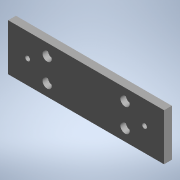
# Autodesk Inventor part: adapter_stage
Saved by Autodesk Inventor 2022 (Build 260153000, 153)
## iProperties
Part Number: adapter_stage
Material: Allgemein
Document SubType Name: Modellieren
Designer: Niclas
Appearance: Vorgabe
Author: Niclas
Autodesk Inventor part; units mm, degrees
ref_plane "YZ-Ebene" through (0, 0, 0) normal (1, 0, 0) x (0, 1, 0)
ref_plane "XZ-Ebene" through (0, 0, 0) normal (0, 1, 0) x (-1, 0, 0)
ref_plane "XY-Ebene" through (0, 0, 0) normal (0, 0, 1) x (1, 0, 0)
sketch "Skizze1" plane through (0, 0, 0) normal (0, 0, 1) x (1, 0, 0)
  line L0 (-200, 60) -> (0, 60)
  line L1 (0, 60) -> (0, 0)
  line L2 (0, 0) -> (-200, 0)
  line L3 (-200, 0) -> (-200, 60)
  dimension "d0" = 200
  dimension "d1" = 60
  constraints: 8 end point, 2 parallel, 1 coincident, 1 horizontal, 1 perpendicular
  measures "d0" distance of L0.start L0.end
  measures "d1" distance of L2.end L0.start
extrude "Extrusion1" add sketch "Skizze1" along normal blind 10
sketch "Skizze2" plane through (0, 0, 10) normal (0, 0, 1) x (1, 0, 0)
  circle A0 centre (-175, 30) radius 3.1
  circle A1 centre (-25, 30) radius 3.1
  line L0 (-200, 0) -> (0, 0) projected
  line L1 (0, 0) -> (0, 60) projected
  circle A2 centre (-150, 45) radius 3.1
  circle A3 centre (-50, 45) radius 3.1
  circle A4 centre (-150, 15) radius 3.1
  circle A5 centre (-50, 15) radius 3.1
  line L2 (0, 60) -> (-200, 60) projected
  dimension "d4" = 6.2
  dimension "d5" = 6.2
  dimension "d6" = 30
  dimension "d7" = 30
  dimension "d8" = 150
  dimension "d9" = 25
  dimension "d10" = 6.2
  dimension "d11" = 6.2
  dimension "d12" = 6.2
  dimension "d13" = 6.2
  dimension "d14" = 30
  dimension "d15" = 30
  dimension "d16" = 100
  dimension "d17" = 100
  dimension "d18" = 50
  dimension "d19" = 50
  dimension "d20" = 15
  dimension "d21" = 15
  constraints: 6 centre point
  measures "d4" diameter of A1
  measures "d5" diameter of A0
  measures "d6" distance from line of A0.centre L0
  measures "d7" distance from line of L0 A1.centre
  measures "d8" distance of A1.centre A0.centre
  measures "d9" distance from line of L1 A1.centre
  measures "d10" diameter of A2
  measures "d11" diameter of A3
  measures "d12" diameter of A5
  measures "d13" diameter of A4
  measures "d14" distance of A4.centre A2.centre
  measures "d15" distance of A5.centre A3.centre
  measures "d16" distance of A5.centre A4.centre
  measures "d17" distance of A3.centre A2.centre
  measures "d18" distance from line of L1 A3.centre
  measures "d19" distance from line of L1 A5.centre
  measures "d20" distance from line of L2 A3.centre
  measures "d21" distance from line of L2 A2.centre
extrude "Extrusion2" cut sketch "Skizze2" against normal blind 15
sketch "Skizze3" plane through (0, 0, 10) normal (0, 0, 1) x (1, 0, 0)
  circle A0 centre (-150, 45) radius 3.1 projected
  circle A1 centre (-150, 45) radius 6
  circle A2 centre (-150, 15) radius 3.1 projected
  circle A3 centre (-150, 15) radius 6
  circle A4 centre (-50, 45) radius 3.1 projected
  circle A5 centre (-50, 15) radius 3.1 projected
  circle A6 centre (-50, 15) radius 6
  circle A7 centre (-50, 45) radius 6
  point P0 (0, 0)
  dimension "d24" = 12
  dimension "d25" = 12
  dimension "d26" = 12
  dimension "d27" = 12
  constraints: 4 centre point, 4 coincident
  measures "d24" diameter of A1
  measures "d25" diameter of A3
  measures "d26" diameter of A6
  measures "d27" diameter of A7
extrude "Extrusion3" cut sketch "Skizze3" against normal blind 7 contours A1 | A3 | A5 | A6 | A7
sketch "Skizze4" plane through (0, 0, 0) normal (0, 0, -1) x (-1, 0, 0)
  circle A0 centre (175, 30) radius 3.1 projected
  circle A1 centre (175, 30) radius 6
  circle A2 centre (25, 30) radius 3.1 projected
  circle A3 centre (25, 30) radius 6
  point P0 (0, 0)
  dimension "d30" = 12
  dimension "d31" = 12
  constraints: 2 centre point, 2 coincident
  measures "d30" diameter of A1
  measures "d31" diameter of A3
extrude "Extrusion4" cut sketch "Skizze4" against normal blind 7 contours A0 | A1 | A2 | A3
